Autodesk Fusion 360 part; units mm, degrees
(part 5 of 7)
sketch "スケッチ10" plane through (0, 0, 2) normal (0, 0, 1) x (-1, 0, 0)
  spline S0 degree 3 poles (-235, 87.4565) (-235.3871, 87.1804) (-235.7742, 86.9044) (-236.1613, 86.6283) (-236.3242, 86.5122) (-236.4823, 86.3889) (-236.6355, 86.2591) (-237.986, 85.1149) (-238.9085, 83.4814) (-239.6002, 81.6203) (-240.237, 79.9069) (-240.7129, 77.9522) (-241.2668, 76.0817) (-241.6514, 74.7828) (-242.0881, 73.5183) (-242.5, 72.6931) knots -0.056001 -0.056001 -0.056001 -0.056001 0 0 0 0.016893 0.016893 0.016893 0.165823 0.165823 0.165823 0.30293 0.30293 0.30293 0.398144 0.398144 0.398144 0.398144
  spline S1 degree 3 poles (-227.5, 72.6931) (-227.6088, 72.9111) (-227.7208, 73.1603) (-227.8326, 73.4325) (-228.2149, 74.3638) (-228.5808, 75.5389) (-228.9195, 76.7225) (-229.4675, 78.6373) (-229.9554, 80.5733) (-230.6468, 82.2521) (-231.3881, 84.0523) (-232.4048, 85.6057) (-233.8387, 86.6283) (-234.2258, 86.9044) (-234.6129, 87.1804) (-235, 87.4565) knots 0.601856 0.601856 0.601856 0.601856 0.626906 0.626906 0.626906 0.71262 0.71262 0.71262 0.851292 0.851292 0.851292 1 1 1 1.056001 1.056001 1.056001 1.056001
  spline S2 degree 3 poles (-220, 87.4565) (-220.3871, 87.1804) (-220.7742, 86.9044) (-221.1613, 86.6283) (-221.3242, 86.5122) (-221.4823, 86.3889) (-221.6355, 86.2591) (-222.986, 85.1149) (-223.9085, 83.4814) (-224.6002, 81.6203) (-225.237, 79.9069) (-225.7129, 77.9522) (-226.2668, 76.0817) (-226.6514, 74.7828) (-227.0881, 73.5183) (-227.5, 72.6931) knots -0.056001 -0.056001 -0.056001 -0.056001 0 0 0 0.016893 0.016893 0.016893 0.165823 0.165823 0.165823 0.30293 0.30293 0.30293 0.398144 0.398144 0.398144 0.398144
  spline S3 degree 3 poles (-212.5, 72.6931) (-212.6088, 72.9111) (-212.7208, 73.1603) (-212.8326, 73.4325) (-213.2149, 74.3638) (-213.5808, 75.5389) (-213.9195, 76.7225) (-214.4675, 78.6373) (-214.9554, 80.5733) (-215.6468, 82.2521) (-216.3881, 84.0523) (-217.4048, 85.6057) (-218.8387, 86.6283) (-219.2258, 86.9044) (-219.6129, 87.1804) (-220, 87.4565) knots 0.601856 0.601856 0.601856 0.601856 0.626906 0.626906 0.626906 0.71262 0.71262 0.71262 0.851292 0.851292 0.851292 1 1 1 1.056001 1.056001 1.056001 1.056001
  spline S4 degree 3 poles (-205, 87.4565) (-205.3871, 87.1804) (-205.7742, 86.9044) (-206.1613, 86.6283) (-206.3242, 86.5122) (-206.4823, 86.3889) (-206.6355, 86.2591) (-207.986, 85.1149) (-208.9085, 83.4814) (-209.6002, 81.6203) (-210.237, 79.9069) (-210.7129, 77.9522) (-211.2668, 76.0817) (-211.6514, 74.7828) (-212.0881, 73.5183) (-212.5, 72.6931) knots -0.056001 -0.056001 -0.056001 -0.056001 0 0 0 0.016893 0.016893 0.016893 0.165823 0.165823 0.165823 0.30293 0.30293 0.30293 0.398144 0.398144 0.398144 0.398144
  spline S5 degree 3 poles (-197.5, 72.6931) (-197.6088, 72.9111) (-197.7208, 73.1603) (-197.8326, 73.4325) (-198.2149, 74.3638) (-198.5808, 75.5389) (-198.9195, 76.7225) (-199.4675, 78.6373) (-199.9554, 80.5733) (-200.6468, 82.2521) (-201.3881, 84.0523) (-202.4048, 85.6057) (-203.8387, 86.6283) (-204.2258, 86.9044) (-204.6129, 87.1804) (-205, 87.4565) knots 0.601856 0.601856 0.601856 0.601856 0.626906 0.626906 0.626906 0.71262 0.71262 0.71262 0.851292 0.851292 0.851292 1 1 1 1.056001 1.056001 1.056001 1.056001
  spline S6 degree 3 poles (-190, 87.4565) (-190.3871, 87.1804) (-190.7742, 86.9044) (-191.1613, 86.6283) (-191.3242, 86.5122) (-191.4823, 86.3889) (-191.6355, 86.2591) (-192.986, 85.1149) (-193.9085, 83.4814) (-194.6002, 81.6203) (-195.237, 79.9069) (-195.7129, 77.9522) (-196.2668, 76.0817) (-196.6514, 74.7828) (-197.0881, 73.5183) (-197.5, 72.6931) knots -0.056001 -0.056001 -0.056001 -0.056001 0 0 0 0.016893 0.016893 0.016893 0.165823 0.165823 0.165823 0.30293 0.30293 0.30293 0.398144 0.398144 0.398144 0.398144
  spline S7 degree 3 poles (-182.5, 72.6931) (-182.6088, 72.9111) (-182.7208, 73.1603) (-182.8326, 73.4325) (-183.2149, 74.3638) (-183.5808, 75.5389) (-183.9195, 76.7225) (-184.4675, 78.6373) (-184.9554, 80.5733) (-185.6468, 82.2521) (-186.3881, 84.0523) (-187.4048, 85.6057) (-188.8387, 86.6283) (-189.2258, 86.9044) (-189.6129, 87.1804) (-190, 87.4565) knots 0.601856 0.601856 0.601856 0.601856 0.626906 0.626906 0.626906 0.71262 0.71262 0.71262 0.851292 0.851292 0.851292 1 1 1 1.056001 1.056001 1.056001 1.056001
  spline S8 degree 3 poles (-175, 87.4565) (-175.3871, 87.1804) (-175.7742, 86.9044) (-176.1613, 86.6283) (-176.3242, 86.5122) (-176.4823, 86.3889) (-176.6355, 86.2591) (-177.986, 85.1149) (-178.9085, 83.4814) (-179.6002, 81.6203) (-180.237, 79.9069) (-180.7129, 77.9522) (-181.2668, 76.0817) (-181.6514, 74.7828) (-182.0881, 73.5183) (-182.5, 72.6931) knots -0.056001 -0.056001 -0.056001 -0.056001 0 0 0 0.016893 0.016893 0.016893 0.165823 0.165823 0.165823 0.30293 0.30293 0.30293 0.398144 0.398144 0.398144 0.398144
  spline S9 degree 3 poles (-167.5, 72.6931) (-167.6088, 72.9111) (-167.7208, 73.1603) (-167.8326, 73.4325) (-168.2149, 74.3638) (-168.5808, 75.5389) (-168.9195, 76.7225) (-169.4675, 78.6373) (-169.9554, 80.5733) (-170.6468, 82.2521) (-171.3881, 84.0523) (-172.4048, 85.6057) (-173.8387, 86.6283) (-174.2258, 86.9044) (-174.6129, 87.1804) (-175, 87.4565) knots 0.601856 0.601856 0.601856 0.601856 0.626906 0.626906 0.626906 0.71262 0.71262 0.71262 0.851292 0.851292 0.851292 1 1 1 1.056001 1.056001 1.056001 1.056001
  spline S10 degree 3 poles (-160, 87.4565) (-160.3871, 87.1804) (-160.7742, 86.9044) (-161.1613, 86.6283) (-161.3242, 86.5122) (-161.4823, 86.3889) (-161.6355, 86.2591) (-162.986, 85.1149) (-163.9085, 83.4814) (-164.6002, 81.6203) (-165.237, 79.9069) (-165.7129, 77.9522) (-166.2668, 76.0817) (-166.6514, 74.7828) (-167.0881, 73.5183) (-167.5, 72.6931) knots -0.056001 -0.056001 -0.056001 -0.056001 0 0 0 0.016893 0.016893 0.016893 0.165823 0.165823 0.165823 0.30293 0.30293 0.30293 0.398144 0.398144 0.398144 0.398144
  spline S11 degree 3 poles (-152.5, 72.6931) (-152.6088, 72.9111) (-152.7208, 73.1603) (-152.8326, 73.4325) (-153.2149, 74.3638) (-153.5808, 75.5389) (-153.9195, 76.7225) (-154.4675, 78.6373) (-154.9554, 80.5733) (-155.6468, 82.2521) (-156.3881, 84.0523) (-157.4048, 85.6057) (-158.8387, 86.6283) (-159.2258, 86.9044) (-159.6129, 87.1804) (-160, 87.4565) knots 0.601856 0.601856 0.601856 0.601856 0.626906 0.626906 0.626906 0.71262 0.71262 0.71262 0.851292 0.851292 0.851292 1 1 1 1.056001 1.056001 1.056001 1.056001
  spline S12 degree 3 poles (-145, 87.4565) (-145.3871, 87.1804) (-145.7742, 86.9044) (-146.1613, 86.6283) (-146.3242, 86.5122) (-146.4823, 86.3889) (-146.6355, 86.2591) (-147.986, 85.1149) (-148.9085, 83.4814) (-149.6002, 81.6203) (-150.237, 79.9069) (-150.7129, 77.9522) (-151.2668, 76.0817) (-151.6514, 74.7828) (-152.0881, 73.5183) (-152.5, 72.6931) knots -0.056001 -0.056001 -0.056001 -0.056001 0 0 0 0.016893 0.016893 0.016893 0.165823 0.165823 0.165823 0.30293 0.30293 0.30293 0.398144 0.398144 0.398144 0.398144
  spline S13 degree 3 poles (-137.5, 72.6931) (-137.6088, 72.9111) (-137.7208, 73.1603) (-137.8326, 73.4325) (-138.2149, 74.3638) (-138.5808, 75.5389) (-138.9195, 76.7225) (-139.4675, 78.6373) (-139.9554, 80.5733) (-140.6468, 82.2521) (-141.3881, 84.0523) (-142.4048, 85.6057) (-143.8387, 86.6283) (-144.2258, 86.9044) (-144.6129, 87.1804) (-145, 87.4565) knots 0.601856 0.601856 0.601856 0.601856 0.626906 0.626906 0.626906 0.71262 0.71262 0.71262 0.851292 0.851292 0.851292 1 1 1 1.056001 1.056001 1.056001 1.056001
  spline S14 degree 3 poles (-130, 87.4565) (-130.3871, 87.1804) (-130.7742, 86.9044) (-131.1613, 86.6283) (-131.3242, 86.5122) (-131.4823, 86.3889) (-131.6355, 86.2591) (-132.986, 85.1149) (-133.9085, 83.4814) (-134.6002, 81.6203) (-135.237, 79.9069) (-135.7129, 77.9522) (-136.2668, 76.0817) (-136.6514, 74.7828) (-137.0881, 73.5183) (-137.5, 72.6931) knots -0.056001 -0.056001 -0.056001 -0.056001 0 0 0 0.016893 0.016893 0.016893 0.165823 0.165823 0.165823 0.30293 0.30293 0.30293 0.398144 0.398144 0.398144 0.398144
  spline S15 degree 3 poles (-122.5, 72.6931) (-122.6088, 72.9111) (-122.7208, 73.1603) (-122.8326, 73.4325) (-123.2149, 74.3638) (-123.5808, 75.5389) (-123.9195, 76.7225) (-124.4675, 78.6373) (-124.9554, 80.5733) (-125.6468, 82.2521) (-126.3881, 84.0523) (-127.4048, 85.6057) (-128.8387, 86.6283) (-129.2258, 86.9044) (-129.6129, 87.1804) (-130, 87.4565) knots 0.601856 0.601856 0.601856 0.601856 0.626906 0.626906 0.626906 0.71262 0.71262 0.71262 0.851292 0.851292 0.851292 1 1 1 1.056001 1.056001 1.056001 1.056001
  spline S16 degree 3 poles (-115, 87.4565) (-115.3871, 87.1804) (-115.7742, 86.9044) (-116.1613, 86.6283) (-116.3242, 86.5122) (-116.4823, 86.3889) (-116.6355, 86.2591) (-117.986, 85.1149) (-118.9085, 83.4814) (-119.6002, 81.6203) (-120.237, 79.9069) (-120.7129, 77.9522) (-121.2668, 76.0817) (-121.6514, 74.7828) (-122.0881, 73.5183) (-122.5, 72.6931) knots -0.056001 -0.056001 -0.056001 -0.056001 0 0 0 0.016893 0.016893 0.016893 0.165823 0.165823 0.165823 0.30293 0.30293 0.30293 0.398144 0.398144 0.398144 0.398144
  spline S17 degree 3 poles (-107.5, 72.6931) (-107.6088, 72.9111) (-107.7208, 73.1603) (-107.8326, 73.4325) (-108.2149, 74.3638) (-108.5808, 75.5389) (-108.9195, 76.7225) (-109.4675, 78.6373) (-109.9554, 80.5733) (-110.6468, 82.2521) (-111.3881, 84.0523) (-112.4048, 85.6057) (-113.8387, 86.6283) (-114.2258, 86.9044) (-114.6129, 87.1804) (-115, 87.4565) knots 0.601856 0.601856 0.601856 0.601856 0.626906 0.626906 0.626906 0.71262 0.71262 0.71262 0.851292 0.851292 0.851292 1 1 1 1.056001 1.056001 1.056001 1.056001
  spline S18 degree 3 poles (-100, 87.4565) (-100.3871, 87.1804) (-100.7742, 86.9044) (-101.1613, 86.6283) (-101.3242, 86.5122) (-101.4823, 86.3889) (-101.6355, 86.2591) (-102.986, 85.1149) (-103.9085, 83.4814) (-104.6002, 81.6203) (-105.237, 79.9069) (-105.7129, 77.9522) (-106.2668, 76.0817) (-106.6514, 74.7828) (-107.0881, 73.5183) (-107.5, 72.6931) knots -0.056001 -0.056001 -0.056001 -0.056001 0 0 0 0.016893 0.016893 0.016893 0.165823 0.165823 0.165823 0.30293 0.30293 0.30293 0.398144 0.398144 0.398144 0.398144
  spline S19 degree 3 poles (-92.5, 72.6931) (-92.6088, 72.9111) (-92.7208, 73.1603) (-92.8326, 73.4325) (-93.2149, 74.3638) (-93.5808, 75.5389) (-93.9195, 76.7225) (-94.4675, 78.6373) (-94.9554, 80.5733) (-95.6468, 82.2521) (-96.3881, 84.0523) (-97.4048, 85.6057) (-98.8387, 86.6283) (-99.2258, 86.9044) (-99.6129, 87.1804) (-100, 87.4565) knots 0.601856 0.601856 0.601856 0.601856 0.626906 0.626906 0.626906 0.71262 0.71262 0.71262 0.851292 0.851292 0.851292 1 1 1 1.056001 1.056001 1.056001 1.056001
  spline S20 degree 3 poles (-85, 87.4565) (-85.3871, 87.1804) (-85.7742, 86.9044) (-86.1613, 86.6283) (-86.3242, 86.5122) (-86.4823, 86.3889) (-86.6355, 86.2591) (-87.986, 85.1149) (-88.9085, 83.4814) (-89.6002, 81.6203) (-90.237, 79.9069) (-90.7129, 77.9522) (-91.2668, 76.0817) (-91.6514, 74.7828) (-92.0881, 73.5183) (-92.5, 72.6931) knots -0.056001 -0.056001 -0.056001 -0.056001 0 0 0 0.016893 0.016893 0.016893 0.165823 0.165823 0.165823 0.30293 0.30293 0.30293 0.398144 0.398144 0.398144 0.398144
  spline S21 degree 3 poles (-77.5, 72.6931) (-77.6088, 72.9111) (-77.7208, 73.1603) (-77.8326, 73.4325) (-78.2149, 74.3638) (-78.5808, 75.5389) (-78.9195, 76.7225) (-79.4675, 78.6373) (-79.9554, 80.5733) (-80.6468, 82.2521) (-81.3881, 84.0523) (-82.4048, 85.6057) (-83.8387, 86.6283) (-84.2258, 86.9044) (-84.6129, 87.1804) (-85, 87.4565) knots 0.601856 0.601856 0.601856 0.601856 0.626906 0.626906 0.626906 0.71262 0.71262 0.71262 0.851292 0.851292 0.851292 1 1 1 1.056001 1.056001 1.056001 1.056001
  spline S22 degree 3 poles (-70, 87.4565) (-70.3871, 87.1804) (-70.7742, 86.9044) (-71.1613, 86.6283) (-71.3242, 86.5122) (-71.4823, 86.3889) (-71.6355, 86.2591) (-72.986, 85.1149) (-73.9085, 83.4814) (-74.6002, 81.6203) (-75.237, 79.9069) (-75.7129, 77.9522) (-76.2668, 76.0817) (-76.6514, 74.7828) (-77.0881, 73.5183) (-77.5, 72.6931) knots -0.056001 -0.056001 -0.056001 -0.056001 0 0 0 0.016893 0.016893 0.016893 0.165823 0.165823 0.165823 0.30293 0.30293 0.30293 0.398144 0.398144 0.398144 0.398144
  spline S23 degree 3 poles (-62.5, 72.6931) (-62.6088, 72.9111) (-62.7208, 73.1603) (-62.8326, 73.4325) (-63.2149, 74.3638) (-63.5808, 75.5389) (-63.9195, 76.7225) (-64.4675, 78.6373) (-64.9554, 80.5733) (-65.6468, 82.2521) (-66.3881, 84.0523) (-67.4048, 85.6057) (-68.8387, 86.6283) (-69.2258, 86.9044) (-69.6129, 87.1804) (-70, 87.4565) knots 0.601856 0.601856 0.601856 0.601856 0.626906 0.626906 0.626906 0.71262 0.71262 0.71262 0.851292 0.851292 0.851292 1 1 1 1.056001 1.056001 1.056001 1.056001
  spline S24 degree 3 poles (-55, 87.4565) (-55.3871, 87.1804) (-55.7742, 86.9044) (-56.1613, 86.6283) (-56.3242, 86.5122) (-56.4823, 86.3889) (-56.6355, 86.2591) (-57.986, 85.1149) (-58.9085, 83.4814) (-59.6002, 81.6203) (-60.237, 79.9069) (-60.7129, 77.9522) (-61.2668, 76.0817) (-61.6514, 74.7828) (-62.0881, 73.5183) (-62.5, 72.6931) knots -0.056001 -0.056001 -0.056001 -0.056001 0 0 0 0.016893 0.016893 0.016893 0.165823 0.165823 0.165823 0.30293 0.30293 0.30293 0.398144 0.398144 0.398144 0.398144
  spline S25 degree 3 poles (-47.5, 72.6931) (-47.6088, 72.9111) (-47.7208, 73.1603) (-47.8326, 73.4325) (-48.2149, 74.3638) (-48.5808, 75.5389) (-48.9195, 76.7225) (-49.4675, 78.6373) (-49.9554, 80.5733) (-50.6468, 82.2521) (-51.3881, 84.0523) (-52.4048, 85.6057) (-53.8387, 86.6283) (-54.2258, 86.9044) (-54.6129, 87.1804) (-55, 87.4565) knots 0.601856 0.601856 0.601856 0.601856 0.626906 0.626906 0.626906 0.71262 0.71262 0.71262 0.851292 0.851292 0.851292 1 1 1 1.056001 1.056001 1.056001 1.056001
  spline S26 degree 3 poles (-40, 87.4565) (-40.3871, 87.1804) (-40.7742, 86.9044) (-41.1613, 86.6283) (-41.3242, 86.5122) (-41.4823, 86.3889) (-41.6355, 86.2591) (-42.986, 85.1149) (-43.9085, 83.4814) (-44.6002, 81.6203) (-45.237, 79.9069) (-45.7129, 77.9522) (-46.2668, 76.0817) (-46.6514, 74.7828) (-47.0881, 73.5183) (-47.5, 72.6931) knots -0.056001 -0.056001 -0.056001 -0.056001 0 0 0 0.016893 0.016893 0.016893 0.165823 0.165823 0.165823 0.30293 0.30293 0.30293 0.398144 0.398144 0.398144 0.398144
  spline S27 degree 3 poles (-32.5, 72.6931) (-32.6088, 72.9111) (-32.7208, 73.1603) (-32.8326, 73.4325) (-33.2149, 74.3638) (-33.5808, 75.5389) (-33.9195, 76.7225) (-34.4675, 78.6373) (-34.9554, 80.5733) (-35.6468, 82.2521) (-36.3881, 84.0523) (-37.4048, 85.6057) (-38.8387, 86.6283) (-39.2258, 86.9044) (-39.6129, 87.1804) (-40, 87.4565) knots 0.601856 0.601856 0.601856 0.601856 0.626906 0.626906 0.626906 0.71262 0.71262 0.71262 0.851292 0.851292 0.851292 1 1 1 1.056001 1.056001 1.056001 1.056001
  spline S28 degree 3 poles (-25, 87.4565) (-25.3871, 87.1804) (-25.7742, 86.9044) (-26.1613, 86.6283) (-26.3242, 86.5122) (-26.4823, 86.3889) (-26.6355, 86.2591) (-27.986, 85.1149) (-28.9085, 83.4814) (-29.6002, 81.6203) (-30.237, 79.9069) (-30.7129, 77.9522) (-31.2668, 76.0817) (-31.6514, 74.7828) (-32.0881, 73.5183) (-32.5, 72.6931) knots -0.056001 -0.056001 -0.056001 -0.056001 0 0 0 0.016893 0.016893 0.016893 0.165823 0.165823 0.165823 0.30293 0.30293 0.30293 0.398144 0.398144 0.398144 0.398144
  spline S29 degree 3 poles (-17.5, 72.6931) (-17.6088, 72.9111) (-17.7208, 73.1603) (-17.8326, 73.4325) (-18.2149, 74.3638) (-18.5808, 75.5389) (-18.9195, 76.7225) (-19.4675, 78.6373) (-19.9554, 80.5733) (-20.6468, 82.2521) (-21.3881, 84.0523) (-22.4048, 85.6057) (-23.8387, 86.6283) (-24.2258, 86.9044) (-24.6129, 87.1804) (-25, 87.4565) knots 0.601856 0.601856 0.601856 0.601856 0.626906 0.626906 0.626906 0.71262 0.71262 0.71262 0.851292 0.851292 0.851292 1 1 1 1.056001 1.056001 1.056001 1.056001
  spline S30 degree 3 poles (-13.2077, 84.4547) (-13.7647, 83.609) (-14.2177, 82.6495) (-14.6002, 81.6203) (-15.237, 79.9069) (-15.7129, 77.9522) (-16.2668, 76.0817) (-16.6514, 74.7828) (-17.0881, 73.5183) (-17.5, 72.6931) knots 0.083469 0.083469 0.083469 0.083469 0.165823 0.165823 0.165823 0.30293 0.30293 0.30293 0.398144 0.398144 0.398144 0.398144
  arc A0 (-17.4992, 87.5) -> (-13.2077, 84.4547) centre (-12.5, 89.9985) ccw
  line L0 (-17.4992, 87.5) -> (-20.5, 87.5)
  arc A1 (-20.5, 97) -> (-20.5, 87.5) centre (-20.5, 92.25) ccw
  line L1 (-20.5, 97) -> (-239.5, 97)
  arc A2 (-239.4991, 87.4565) -> (-239.5, 97) centre (-239.547, 92.2282) ccw
  line L2 (-239.4991, 87.4565) -> (-242.5226, 87.4565)
  arc A3 (-246.7932, 84.4545) -> (-242.5226, 87.4565) centre (-247.5, 89.9985) ccw
  spline S31 degree 3 poles (-242.5, 72.6931) (-242.6088, 72.9111) (-242.7208, 73.1603) (-242.8326, 73.4325) (-243.2149, 74.3638) (-243.5808, 75.5389) (-243.9195, 76.7225) (-244.4675, 78.6373) (-244.9554, 80.5733) (-245.6468, 82.2521) (-245.9719, 83.0417) (-246.3501, 83.7838) (-246.7932, 84.4545) knots 0.601856 0.601856 0.601856 0.601856 0.626906 0.626906 0.626906 0.71262 0.71262 0.71262 0.851292 0.851292 0.851292 0.916519 0.916519 0.916519 0.916519
  line L3 (-39.8743, 92) -> (-220.0824, 92)
  spline S32 degree 5 poles (-25.25, 97) (-25.4197, 97) (-25.7703, 96.9623) (-26.3295, 96.7927) (-27.1433, 96.3615) (-28.2841, 95.5945) (-29.5597, 94.7356) (-30.9794, 93.9127) (-32.5405, 93.2057) (-34.2322, 92.6511) (-36.0421, 92.261) (-37.5756, 92.0789) (-38.7706, 92.0126) (-39.5869, 91.9991) (-40, 92) knots 0 0 0 0 0 0 0.1 0.2 0.3 0.4 0.5 0.6 0.7 0.8 0.9 1 1 1 1 1 1
  spline S33 degree 5 poles (-234.7751, 97) (-234.578, 97) (-234.181, 96.9624) (-233.577, 96.7931) (-232.7489, 96.3627) (-231.6433, 95.5968) (-230.4283, 94.7389) (-229.0695, 93.9166) (-227.5527, 93.2097) (-225.8807, 92.6548) (-224.0629, 92.2639) (-222.5008, 92.0808) (-221.2722, 92.0136) (-220.4282, 91.9994) (-220, 92) knots 0 0 0 0 0 0 0.1 0.2 0.3 0.4 0.5 0.6 0.7 0.8 0.9 1 1 1 1 1 1
  line L4 (-236, 97) -> (-233.5501, 97)
  line L5 (-24.1934, 97) -> (-26.3066, 97)
  point P0 (-30, 94.5)
  point P1 (-230, 94.5)
  constraint coincident L1 S32.start
  constraint coincident L3 S32.end
  constraint coincident L1 S33.start
  constraint coincident L3 S33.end
  constraint midpoint S33.start L4
  constraint coincident L1 L4.start
  constraint midpoint S32.start L5
  constraint coincident L1 L5.start
  constraint coincident S32 L3.start
  constraint coincident S33 L3.end
sketch "スケッチ11" plane through (0, 0, 2) normal (0, 0, 1) x (-1, 0, 0)
  spline S0 degree 5 poles (-25.25, 97) (-25.4197, 97) (-25.7703, 96.9623) (-26.3295, 96.7927) (-27.1433, 96.3615) (-28.2841, 95.5945) (-29.5597, 94.7356) (-30.9794, 93.9127) (-32.5405, 93.2057) (-34.2322, 92.6511) (-36.0201, 92.2658) (-37.5289, 92.0845) (-38.6979, 92.0167) (-39.4875, 92.0009) (-39.8743, 92) knots 0 0 0 0 0 0 0.1 0.2 0.3 0.4 0.5 0.6 0.7 0.8 0.9 0.993905 0.993905 0.993905 0.993905 0.993905 0.993905
  line L0 (-39.8743, 92) -> (-220.0824, 92)
  spline S1 degree 5 poles (-234.7751, 97) (-234.578, 97) (-234.181, 96.9624) (-233.577, 96.7931) (-232.7489, 96.3627) (-231.6433, 95.5968) (-230.4283, 94.7389) (-229.0695, 93.9166) (-227.5527, 93.2097) (-225.8807, 92.6548) (-224.0769, 92.2669) (-222.5308, 92.0843) (-221.3195, 92.0162) (-220.4932, 92.0006) (-220.0824, 92) knots 0 0 0 0 0 0 0.1 0.2 0.3 0.4 0.5 0.6 0.7 0.8 0.9 0.99615 0.99615 0.99615 0.99615 0.99615 0.99615
  line L1 (-234.7751, 97) -> (-239.5, 97)
  arc A0 (-239.4991, 87.4565) -> (-239.5, 97) centre (-239.547, 92.2282) ccw
  line L2 (-239.4991, 87.4565) -> (-242.5226, 87.4565)
  arc A1 (-246.7932, 84.4545) -> (-242.5226, 87.4565) centre (-247.5, 89.9985) ccw
  spline S2 degree 3 poles (-242.5, 72.6931) (-242.6088, 72.9111) (-242.7208, 73.1603) (-242.8326, 73.4325) (-243.2149, 74.3638) (-243.5808, 75.5389) (-243.9195, 76.7225) (-244.4675, 78.6373) (-244.9554, 80.5733) (-245.6468, 82.2521) (-245.9719, 83.0417) (-246.3501, 83.7838) (-246.7932, 84.4545) knots 0.601856 0.601856 0.601856 0.601856 0.626906 0.626906 0.626906 0.71262 0.71262 0.71262 0.851292 0.851292 0.851292 0.916519 0.916519 0.916519 0.916519
  spline S3 degree 3 poles (-235, 87.4565) (-235.3871, 87.1804) (-235.7742, 86.9044) (-236.1613, 86.6283) (-236.3242, 86.5122) (-236.4823, 86.3889) (-236.6355, 86.2591) (-237.986, 85.1149) (-238.9085, 83.4814) (-239.6002, 81.6203) (-240.237, 79.9069) (-240.7129, 77.9522) (-241.2668, 76.0817) (-241.6514, 74.7828) (-242.0881, 73.5183) (-242.5, 72.6931) knots -0.056001 -0.056001 -0.056001 -0.056001 0 0 0 0.016893 0.016893 0.016893 0.165823 0.165823 0.165823 0.30293 0.30293 0.30293 0.398144 0.398144 0.398144 0.398144
  spline S4 degree 3 poles (-227.5, 72.6931) (-227.6088, 72.9111) (-227.7208, 73.1603) (-227.8326, 73.4325) (-228.2149, 74.3638) (-228.5808, 75.5389) (-228.9195, 76.7225) (-229.4675, 78.6373) (-229.9554, 80.5733) (-230.6468, 82.2521) (-231.3881, 84.0523) (-232.4048, 85.6057) (-233.8387, 86.6283) (-234.2258, 86.9044) (-234.6129, 87.1804) (-235, 87.4565) knots 0.601856 0.601856 0.601856 0.601856 0.626906 0.626906 0.626906 0.71262 0.71262 0.71262 0.851292 0.851292 0.851292 1 1 1 1.056001 1.056001 1.056001 1.056001
  spline S5 degree 3 poles (-220, 87.4565) (-220.3871, 87.1804) (-220.7742, 86.9044) (-221.1613, 86.6283) (-221.3242, 86.5122) (-221.4823, 86.3889) (-221.6355, 86.2591) (-222.986, 85.1149) (-223.9085, 83.4814) (-224.6002, 81.6203) (-225.237, 79.9069) (-225.7129, 77.9522) (-226.2668, 76.0817) (-226.6514, 74.7828) (-227.0881, 73.5183) (-227.5, 72.6931) knots -0.056001 -0.056001 -0.056001 -0.056001 0 0 0 0.016893 0.016893 0.016893 0.165823 0.165823 0.165823 0.30293 0.30293 0.30293 0.398144 0.398144 0.398144 0.398144
  spline S6 degree 3 poles (-212.5, 72.6931) (-212.6088, 72.9111) (-212.7208, 73.1603) (-212.8326, 73.4325) (-213.2149, 74.3638) (-213.5808, 75.5389) (-213.9195, 76.7225) (-214.4675, 78.6373) (-214.9554, 80.5733) (-215.6468, 82.2521) (-216.3881, 84.0523) (-217.4048, 85.6057) (-218.8387, 86.6283) (-219.2258, 86.9044) (-219.6129, 87.1804) (-220, 87.4565) knots 0.601856 0.601856 0.601856 0.601856 0.626906 0.626906 0.626906 0.71262 0.71262 0.71262 0.851292 0.851292 0.851292 1 1 1 1.056001 1.056001 1.056001 1.056001
  spline S7 degree 3 poles (-205, 87.4565) (-205.3871, 87.1804) (-205.7742, 86.9044) (-206.1613, 86.6283) (-206.3242, 86.5122) (-206.4823, 86.3889) (-206.6355, 86.2591) (-207.986, 85.1149) (-208.9085, 83.4814) (-209.6002, 81.6203) (-210.237, 79.9069) (-210.7129, 77.9522) (-211.2668, 76.0817) (-211.6514, 74.7828) (-212.0881, 73.5183) (-212.5, 72.6931) knots -0.056001 -0.056001 -0.056001 -0.056001 0 0 0 0.016893 0.016893 0.016893 0.165823 0.165823 0.165823 0.30293 0.30293 0.30293 0.398144 0.398144 0.398144 0.398144
  spline S8 degree 3 poles (-197.5, 72.6931) (-197.6088, 72.9111) (-197.7208, 73.1603) (-197.8326, 73.4325) (-198.2149, 74.3638) (-198.5808, 75.5389) (-198.9195, 76.7225) (-199.4675, 78.6373) (-199.9554, 80.5733) (-200.6468, 82.2521) (-201.3881, 84.0523) (-202.4048, 85.6057) (-203.8387, 86.6283) (-204.2258, 86.9044) (-204.6129, 87.1804) (-205, 87.4565) knots 0.601856 0.601856 0.601856 0.601856 0.626906 0.626906 0.626906 0.71262 0.71262 0.71262 0.851292 0.851292 0.851292 1 1 1 1.056001 1.056001 1.056001 1.056001
  spline S9 degree 3 poles (-190, 87.4565) (-190.3871, 87.1804) (-190.7742, 86.9044) (-191.1613, 86.6283) (-191.3242, 86.5122) (-191.4823, 86.3889) (-191.6355, 86.2591) (-192.986, 85.1149) (-193.9085, 83.4814) (-194.6002, 81.6203) (-195.237, 79.9069) (-195.7129, 77.9522) (-196.2668, 76.0817) (-196.6514, 74.7828) (-197.0881, 73.5183) (-197.5, 72.6931) knots -0.056001 -0.056001 -0.056001 -0.056001 0 0 0 0.016893 0.016893 0.016893 0.165823 0.165823 0.165823 0.30293 0.30293 0.30293 0.398144 0.398144 0.398144 0.398144
  spline S10 degree 3 poles (-182.5, 72.6931) (-182.6088, 72.9111) (-182.7208, 73.1603) (-182.8326, 73.4325) (-183.2149, 74.3638) (-183.5808, 75.5389) (-183.9195, 76.7225) (-184.4675, 78.6373) (-184.9554, 80.5733) (-185.6468, 82.2521) (-186.3881, 84.0523) (-187.4048, 85.6057) (-188.8387, 86.6283) (-189.2258, 86.9044) (-189.6129, 87.1804) (-190, 87.4565) knots 0.601856 0.601856 0.601856 0.601856 0.626906 0.626906 0.626906 0.71262 0.71262 0.71262 0.851292 0.851292 0.851292 1 1 1 1.056001 1.056001 1.056001 1.056001
  spline S11 degree 3 poles (-175, 87.4565) (-175.3871, 87.1804) (-175.7742, 86.9044) (-176.1613, 86.6283) (-176.3242, 86.5122) (-176.4823, 86.3889) (-176.6355, 86.2591) (-177.986, 85.1149) (-178.9085, 83.4814) (-179.6002, 81.6203) (-180.237, 79.9069) (-180.7129, 77.9522) (-181.2668, 76.0817) (-181.6514, 74.7828) (-182.0881, 73.5183) (-182.5, 72.6931) knots -0.056001 -0.056001 -0.056001 -0.056001 0 0 0 0.016893 0.016893 0.016893 0.165823 0.165823 0.165823 0.30293 0.30293 0.30293 0.398144 0.398144 0.398144 0.398144
  spline S12 degree 3 poles (-167.5, 72.6931) (-167.6088, 72.9111) (-167.7208, 73.1603) (-167.8326, 73.4325) (-168.2149, 74.3638) (-168.5808, 75.5389) (-168.9195, 76.7225) (-169.4675, 78.6373) (-169.9554, 80.5733) (-170.6468, 82.2521) (-171.3881, 84.0523) (-172.4048, 85.6057) (-173.8387, 86.6283) (-174.2258, 86.9044) (-174.6129, 87.1804) (-175, 87.4565) knots 0.601856 0.601856 0.601856 0.601856 0.626906 0.626906 0.626906 0.71262 0.71262 0.71262 0.851292 0.851292 0.851292 1 1 1 1.056001 1.056001 1.056001 1.056001
  spline S13 degree 3 poles (-160, 87.4565) (-160.3871, 87.1804) (-160.7742, 86.9044) (-161.1613, 86.6283) (-161.3242, 86.5122) (-161.4823, 86.3889) (-161.6355, 86.2591) (-162.986, 85.1149) (-163.9085, 83.4814) (-164.6002, 81.6203) (-165.237, 79.9069) (-165.7129, 77.9522) (-166.2668, 76.0817) (-166.6514, 74.7828) (-167.0881, 73.5183) (-167.5, 72.6931) knots -0.056001 -0.056001 -0.056001 -0.056001 0 0 0 0.016893 0.016893 0.016893 0.165823 0.165823 0.165823 0.30293 0.30293 0.30293 0.398144 0.398144 0.398144 0.398144
  spline S14 degree 3 poles (-152.5, 72.6931) (-152.6088, 72.9111) (-152.7208, 73.1603) (-152.8326, 73.4325) (-153.2149, 74.3638) (-153.5808, 75.5389) (-153.9195, 76.7225) (-154.4675, 78.6373) (-154.9554, 80.5733) (-155.6468, 82.2521) (-156.3881, 84.0523) (-157.4048, 85.6057) (-158.8387, 86.6283) (-159.2258, 86.9044) (-159.6129, 87.1804) (-160, 87.4565) knots 0.601856 0.601856 0.601856 0.601856 0.626906 0.626906 0.626906 0.71262 0.71262 0.71262 0.851292 0.851292 0.851292 1 1 1 1.056001 1.056001 1.056001 1.056001
  spline S15 degree 3 poles (-145, 87.4565) (-145.3871, 87.1804) (-145.7742, 86.9044) (-146.1613, 86.6283) (-146.3242, 86.5122) (-146.4823, 86.3889) (-146.6355, 86.2591) (-147.986, 85.1149) (-148.9085, 83.4814) (-149.6002, 81.6203) (-150.237, 79.9069) (-150.7129, 77.9522) (-151.2668, 76.0817) (-151.6514, 74.7828) (-152.0881, 73.5183) (-152.5, 72.6931) knots -0.056001 -0.056001 -0.056001 -0.056001 0 0 0 0.016893 0.016893 0.016893 0.165823 0.165823 0.165823 0.30293 0.30293 0.30293 0.398144 0.398144 0.398144 0.398144
  spline S16 degree 3 poles (-137.5, 72.6931) (-137.6088, 72.9111) (-137.7208, 73.1603) (-137.8326, 73.4325) (-138.2149, 74.3638) (-138.5808, 75.5389) (-138.9195, 76.7225) (-139.4675, 78.6373) (-139.9554, 80.5733) (-140.6468, 82.2521) (-141.3881, 84.0523) (-142.4048, 85.6057) (-143.8387, 86.6283) (-144.2258, 86.9044) (-144.6129, 87.1804) (-145, 87.4565) knots 0.601856 0.601856 0.601856 0.601856 0.626906 0.626906 0.626906 0.71262 0.71262 0.71262 0.851292 0.851292 0.851292 1 1 1 1.056001 1.056001 1.056001 1.056001
  spline S17 degree 3 poles (-130, 87.4565) (-130.3871, 87.1804) (-130.7742, 86.9044) (-131.1613, 86.6283) (-131.3242, 86.5122) (-131.4823, 86.3889) (-131.6355, 86.2591) (-132.986, 85.1149) (-133.9085, 83.4814) (-134.6002, 81.6203) (-135.237, 79.9069) (-135.7129, 77.9522) (-136.2668, 76.0817) (-136.6514, 74.7828) (-137.0881, 73.5183) (-137.5, 72.6931) knots -0.056001 -0.056001 -0.056001 -0.056001 0 0 0 0.016893 0.016893 0.016893 0.165823 0.165823 0.165823 0.30293 0.30293 0.30293 0.398144 0.398144 0.398144 0.398144
  spline S18 degree 3 poles (-122.5, 72.6931) (-122.6088, 72.9111) (-122.7208, 73.1603) (-122.8326, 73.4325) (-123.2149, 74.3638) (-123.5808, 75.5389) (-123.9195, 76.7225) (-124.4675, 78.6373) (-124.9554, 80.5733) (-125.6468, 82.2521) (-126.3881, 84.0523) (-127.4048, 85.6057) (-128.8387, 86.6283) (-129.2258, 86.9044) (-129.6129, 87.1804) (-130, 87.4565) knots 0.601856 0.601856 0.601856 0.601856 0.626906 0.626906 0.626906 0.71262 0.71262 0.71262 0.851292 0.851292 0.851292 1 1 1 1.056001 1.056001 1.056001 1.056001
  spline S19 degree 3 poles (-115, 87.4565) (-115.3871, 87.1804) (-115.7742, 86.9044) (-116.1613, 86.6283) (-116.3242, 86.5122) (-116.4823, 86.3889) (-116.6355, 86.2591) (-117.986, 85.1149) (-118.9085, 83.4814) (-119.6002, 81.6203) (-120.237, 79.9069) (-120.7129, 77.9522) (-121.2668, 76.0817) (-121.6514, 74.7828) (-122.0881, 73.5183) (-122.5, 72.6931) knots -0.056001 -0.056001 -0.056001 -0.056001 0 0 0 0.016893 0.016893 0.016893 0.165823 0.165823 0.165823 0.30293 0.30293 0.30293 0.398144 0.398144 0.398144 0.398144
  spline S20 degree 3 poles (-107.5, 72.6931) (-107.6088, 72.9111) (-107.7208, 73.1603) (-107.8326, 73.4325) (-108.2149, 74.3638) (-108.5808, 75.5389) (-108.9195, 76.7225) (-109.4675, 78.6373) (-109.9554, 80.5733) (-110.6468, 82.2521) (-111.3881, 84.0523) (-112.4048, 85.6057) (-113.8387, 86.6283) (-114.2258, 86.9044) (-114.6129, 87.1804) (-115, 87.4565) knots 0.601856 0.601856 0.601856 0.601856 0.626906 0.626906 0.626906 0.71262 0.71262 0.71262 0.851292 0.851292 0.851292 1 1 1 1.056001 1.056001 1.056001 1.056001
  spline S21 degree 3 poles (-100, 87.4565) (-100.3871, 87.1804) (-100.7742, 86.9044) (-101.1613, 86.6283) (-101.3242, 86.5122) (-101.4823, 86.3889) (-101.6355, 86.2591) (-102.986, 85.1149) (-103.9085, 83.4814) (-104.6002, 81.6203) (-105.237, 79.9069) (-105.7129, 77.9522) (-106.2668, 76.0817) (-106.6514, 74.7828) (-107.0881, 73.5183) (-107.5, 72.6931) knots -0.056001 -0.056001 -0.056001 -0.056001 0 0 0 0.016893 0.016893 0.016893 0.165823 0.165823 0.165823 0.30293 0.30293 0.30293 0.398144 0.398144 0.398144 0.398144
  spline S22 degree 3 poles (-92.5, 72.6931) (-92.6088, 72.9111) (-92.7208, 73.1603) (-92.8326, 73.4325) (-93.2149, 74.3638) (-93.5808, 75.5389) (-93.9195, 76.7225) (-94.4675, 78.6373) (-94.9554, 80.5733) (-95.6468, 82.2521) (-96.3881, 84.0523) (-97.4048, 85.6057) (-98.8387, 86.6283) (-99.2258, 86.9044) (-99.6129, 87.1804) (-100, 87.4565) knots 0.601856 0.601856 0.601856 0.601856 0.626906 0.626906 0.626906 0.71262 0.71262 0.71262 0.851292 0.851292 0.851292 1 1 1 1.056001 1.056001 1.056001 1.056001
  spline S23 degree 3 poles (-85, 87.4565) (-85.3871, 87.1804) (-85.7742, 86.9044) (-86.1613, 86.6283) (-86.3242, 86.5122) (-86.4823, 86.3889) (-86.6355, 86.2591) (-87.986, 85.1149) (-88.9085, 83.4814) (-89.6002, 81.6203) (-90.237, 79.9069) (-90.7129, 77.9522) (-91.2668, 76.0817) (-91.6514, 74.7828) (-92.0881, 73.5183) (-92.5, 72.6931) knots -0.056001 -0.056001 -0.056001 -0.056001 0 0 0 0.016893 0.016893 0.016893 0.165823 0.165823 0.165823 0.30293 0.30293 0.30293 0.398144 0.398144 0.398144 0.398144
  spline S24 degree 3 poles (-77.5, 72.6931) (-77.6088, 72.9111) (-77.7208, 73.1603) (-77.8326, 73.4325) (-78.2149, 74.3638) (-78.5808, 75.5389) (-78.9195, 76.7225) (-79.4675, 78.6373) (-79.9554, 80.5733) (-80.6468, 82.2521) (-81.3881, 84.0523) (-82.4048, 85.6057) (-83.8387, 86.6283) (-84.2258, 86.9044) (-84.6129, 87.1804) (-85, 87.4565) knots 0.601856 0.601856 0.601856 0.601856 0.626906 0.626906 0.626906 0.71262 0.71262 0.71262 0.851292 0.851292 0.851292 1 1 1 1.056001 1.056001 1.056001 1.056001
  spline S25 degree 3 poles (-70, 87.4565) (-70.3871, 87.1804) (-70.7742, 86.9044) (-71.1613, 86.6283) (-71.3242, 86.5122) (-71.4823, 86.3889) (-71.6355, 86.2591) (-72.986, 85.1149) (-73.9085, 83.4814) (-74.6002, 81.6203) (-75.237, 79.9069) (-75.7129, 77.9522) (-76.2668, 76.0817) (-76.6514, 74.7828) (-77.0881, 73.5183) (-77.5, 72.6931) knots -0.056001 -0.056001 -0.056001 -0.056001 0 0 0 0.016893 0.016893 0.016893 0.165823 0.165823 0.165823 0.30293 0.30293 0.30293 0.398144 0.398144 0.398144 0.398144
  spline S26 degree 3 poles (-62.5, 72.6931) (-62.6088, 72.9111) (-62.7208, 73.1603) (-62.8326, 73.4325) (-63.2149, 74.3638) (-63.5808, 75.5389) (-63.9195, 76.7225) (-64.4675, 78.6373) (-64.9554, 80.5733) (-65.6468, 82.2521) (-66.3881, 84.0523) (-67.4048, 85.6057) (-68.8387, 86.6283) (-69.2258, 86.9044) (-69.6129, 87.1804) (-70, 87.4565) knots 0.601856 0.601856 0.601856 0.601856 0.626906 0.626906 0.626906 0.71262 0.71262 0.71262 0.851292 0.851292 0.851292 1 1 1 1.056001 1.056001 1.056001 1.056001
  spline S27 degree 3 poles (-55, 87.4565) (-55.3871, 87.1804) (-55.7742, 86.9044) (-56.1613, 86.6283) (-56.3242, 86.5122) (-56.4823, 86.3889) (-56.6355, 86.2591) (-57.986, 85.1149) (-58.9085, 83.4814) (-59.6002, 81.6203) (-60.237, 79.9069) (-60.7129, 77.9522) (-61.2668, 76.0817) (-61.6514, 74.7828) (-62.0881, 73.5183) (-62.5, 72.6931) knots -0.056001 -0.056001 -0.056001 -0.056001 0 0 0 0.016893 0.016893 0.016893 0.165823 0.165823 0.165823 0.30293 0.30293 0.30293 0.398144 0.398144 0.398144 0.398144
  spline S28 degree 3 poles (-47.5, 72.6931) (-47.6088, 72.9111) (-47.7208, 73.1603) (-47.8326, 73.4325) (-48.2149, 74.3638) (-48.5808, 75.5389) (-48.9195, 76.7225) (-49.4675, 78.6373) (-49.9554, 80.5733) (-50.6468, 82.2521) (-51.3881, 84.0523) (-52.4048, 85.6057) (-53.8387, 86.6283) (-54.2258, 86.9044) (-54.6129, 87.1804) (-55, 87.4565) knots 0.601856 0.601856 0.601856 0.601856 0.626906 0.626906 0.626906 0.71262 0.71262 0.71262 0.851292 0.851292 0.851292 1 1 1 1.056001 1.056001 1.056001 1.056001
  spline S29 degree 3 poles (-40, 87.4565) (-40.3871, 87.1804) (-40.7742, 86.9044) (-41.1613, 86.6283) (-41.3242, 86.5122) (-41.4823, 86.3889) (-41.6355, 86.2591) (-42.986, 85.1149) (-43.9085, 83.4814) (-44.6002, 81.6203) (-45.237, 79.9069) (-45.7129, 77.9522) (-46.2668, 76.0817) (-46.6514, 74.7828) (-47.0881, 73.5183) (-47.5, 72.6931) knots -0.056001 -0.056001 -0.056001 -0.056001 0 0 0 0.016893 0.016893 0.016893 0.165823 0.165823 0.165823 0.30293 0.30293 0.30293 0.398144 0.398144 0.398144 0.398144
  spline S30 degree 3 poles (-32.5, 72.6931) (-32.6088, 72.9111) (-32.7208, 73.1603) (-32.8326, 73.4325) (-33.2149, 74.3638) (-33.5808, 75.5389) (-33.9195, 76.7225) (-34.4675, 78.6373) (-34.9554, 80.5733) (-35.6468, 82.2521) (-36.3881, 84.0523) (-37.4048, 85.6057) (-38.8387, 86.6283) (-39.2258, 86.9044) (-39.6129, 87.1804) (-40, 87.4565) knots 0.601856 0.601856 0.601856 0.601856 0.626906 0.626906 0.626906 0.71262 0.71262 0.71262 0.851292 0.851292 0.851292 1 1 1 1.056001 1.056001 1.056001 1.056001
  spline S31 degree 3 poles (-25, 87.4565) (-25.3871, 87.1804) (-25.7742, 86.9044) (-26.1613, 86.6283) (-26.3242, 86.5122) (-26.4823, 86.3889) (-26.6355, 86.2591) (-27.986, 85.1149) (-28.9085, 83.4814) (-29.6002, 81.6203) (-30.237, 79.9069) (-30.7129, 77.9522) (-31.2668, 76.0817) (-31.6514, 74.7828) (-32.0881, 73.5183) (-32.5, 72.6931) knots -0.056001 -0.056001 -0.056001 -0.056001 0 0 0 0.016893 0.016893 0.016893 0.165823 0.165823 0.165823 0.30293 0.30293 0.30293 0.398144 0.398144 0.398144 0.398144
  spline S32 degree 3 poles (-17.5, 72.6931) (-17.6088, 72.9111) (-17.7208, 73.1603) (-17.8326, 73.4325) (-18.2149, 74.3638) (-18.5808, 75.5389) (-18.9195, 76.7225) (-19.4675, 78.6373) (-19.9554, 80.5733) (-20.6468, 82.2521) (-21.3881, 84.0523) (-22.4048, 85.6057) (-23.8387, 86.6283) (-24.2258, 86.9044) (-24.6129, 87.1804) (-25, 87.4565) knots 0.601856 0.601856 0.601856 0.601856 0.626906 0.626906 0.626906 0.71262 0.71262 0.71262 0.851292 0.851292 0.851292 1 1 1 1.056001 1.056001 1.056001 1.056001
  spline S33 degree 3 poles (-13.2077, 84.4547) (-13.7647, 83.609) (-14.2177, 82.6495) (-14.6002, 81.6203) (-15.237, 79.9069) (-15.7129, 77.9522) (-16.2668, 76.0817) (-16.6514, 74.7828) (-17.0881, 73.5183) (-17.5, 72.6931) knots 0.083469 0.083469 0.083469 0.083469 0.165823 0.165823 0.165823 0.30293 0.30293 0.30293 0.398144 0.398144 0.398144 0.398144
  arc A2 (-17.4992, 87.5) -> (-13.2077, 84.4547) centre (-12.5, 89.9985) ccw
  line L3 (-17.4992, 87.5) -> (-20.5, 87.5)
  arc A3 (-20.5, 97) -> (-20.5, 87.5) centre (-20.5, 92.25) ccw
  line L4 (-20.5, 97) -> (-25.25, 97)
  line L5 (-22.8584, 88.1269) -> (-23.7547, 86.5675)
  line L6 (-236.2453, 86.5675) -> (-237.1076, 88.1269)
  constraint coincident A3 L5.start
  constraint coincident S32 L5.end
  constraint coincident S3 L6.start
  constraint coincident A0 L6.end
sketch "スケッチ12" plane through (0, 0, 0) normal (0, 0, 1) x (1, 0, 0)